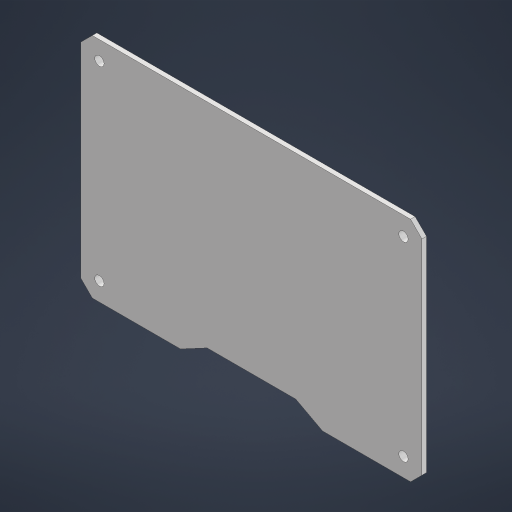
# Autodesk Inventor part: Top
Saved by Autodesk Inventor 2024.2 (Build 282272000, 272)
## iProperties
Created: 2024-06-04
Part Number: Top
Material: Generic
Document SubType Name: Modeling
Designer: simon
Density: 1 g/cm^3
Appearance: Default
Author: simon
Autodesk Inventor part; units mm, degrees
ref_plane "YZ Plane" through (0, 0, 0) normal (1, 0, 0) x (0, 1, 0)
ref_plane "XZ Plane" through (0, 0, 0) normal (0, 1, 0) x (-1, 0, 0)
ref_plane "XY Plane" through (0, 0, 0) normal (0, 0, 1) x (1, 0, 0)
sketch "Sketch1" plane through (0, 0, 0) normal (0, 0, 1) x (1, 0, 0)
  line L0 (0, 0) -> (120, 0)
  line L1 (120, 0) -> (120, 80)
  line L2 (120, 80) -> (0, 80)
  line L3 (0, 80) -> (0, 0)
  line L4 (114.4, 1.6) -> (85, 1.6) projected
  line L5 (75.6, 6.6) -> (85, 1.6) projected
  line L6 (44.4, 6.6) -> (75.6, 6.6) projected
  line L7 (35, 1.6) -> (44.4, 6.6) projected
  line L8 (35, 1.6) -> (5.6, 1.6) projected
  line L9 (1.6, 5.6) -> (5.6, 1.6) projected
  line L10 (1.6, 5.6) -> (1.6, 74.4) projected
  line L11 (5.6, 78.4) -> (1.6, 74.4) projected
  line L12 (5.6, 78.4) -> (114.4, 78.4) projected
  line L13 (118.4, 74.4) -> (114.4, 78.4) projected
  line L14 (118.4, 74.4) -> (118.4, 5.6) projected
  line L15 (114.4, 1.6) -> (118.4, 5.6) projected
  line L16 (116, 80) -> (120, 76) projected
  line L17 (116, 80) -> (4, 80) projected
  line L18 (0, 76) -> (4, 80) projected
  line L19 (0, 76) -> (0, 4) projected
  line L20 (4, 0) -> (0, 4) projected
  line L21 (4, 0) -> (35, 0) projected
  line L22 (44.4, 5) -> (35, 0) projected
  line L23 (44.4, 5) -> (75.6, 5) projected
  line L24 (75.6, 5) -> (85, 0) projected
  line L25 (85, 0) -> (116, 0) projected
  line L26 (120, 4) -> (116, 0) projected
  line L27 (120, 4) -> (120, 76) projected
  circle A0 centre (6.5, 73.5) radius 2 projected
  circle A1 centre (6.5, 6.5) radius 2 projected
  circle A2 centre (113.5, 6.5) radius 2 projected
  circle A3 centre (113.5, 73.5) radius 2 projected
  circle A4 centre (6.5, 73.5) radius 1.65
  circle A5 centre (113.5, 73.5) radius 1.65
  circle A6 centre (113.5, 6.5) radius 1.65
  circle A7 centre (6.5, 6.5) radius 1.65
  line L28 (0, 4) -> (4, 0)
  line L29 (0, 76) -> (4, 80)
  line L30 (116, 80) -> (120, 76)
  line L31 (116, 0) -> (120, 4)
  line L32 (35, 0) -> (44.4, 5)
  line L33 (44.4, 5) -> (75.6, 5)
  line L34 (75.6, 5) -> (85, 0)
  dimension "d0" = 120
  dimension "d1" = 80
  dimension "d4" = 3.3
  dimension "d5" = 3.3
  dimension "d6" = 3.3
  dimension "d7" = 3.3
  constraints: 22 end point, 7 equal length, 4 centre point, 4 coincident, 2 perpendicular, 1 horizontal, 1 point on line
  measures "d0" distance of L2.end L1.end
  measures "d1" distance of L1.end L0.end
  measures "d4" diameter of A4
  measures "d5" diameter of A5
  measures "d6" diameter of A6
  measures "d7" diameter of A7
extrude "Extrusion1" add sketch "Sketch1" along normal blind 1.6 contours L20 L3 L18 L2 L16 L1 L26 L0 L24 L23 L22 | L4 L5 L6 L7 L8 L9 L10 L11 L12 L13 L14 L15 | A0 | A1 | A2 | A3
sketch "Sketch2" plane through (0, 0, 1.6) normal (0, 0, 1) x (1, 0, 0)
  line L0 (5.6, 78.4) -> (114.4, 78.4) projected
  line L1 (5.6, 78.4) -> (1.6, 74.4) projected
  line L2 (1.6, 5.6) -> (1.6, 74.4) projected
  circle A0 centre (6.5, 73.5) radius 2 projected
  circle A1 centre (6.5, 6.5) radius 2 projected
  line L3 (1.6, 5.6) -> (5.6, 1.6) projected
  line L4 (16.9137, 1.6) -> (1.6, 16.9137) projected
  line L5 (35, 1.6) -> (5.6, 1.6) projected
  line L6 (35, 1.6) -> (44.4, 6.6) projected
  line L7 (44.4, 6.6) -> (75.6, 6.6) projected
  line L8 (75.6, 6.6) -> (85, 1.6) projected
  line L9 (114.4, 1.6) -> (85, 1.6) projected
  line L10 (114.4, 1.6) -> (118.4, 5.6) projected
  line L11 (118.4, 74.4) -> (118.4, 5.6) projected
  line L12 (118.4, 16.9137) -> (103.0863, 1.6) projected
  circle A2 centre (113.5, 6.5) radius 2 projected
  line L13 (103.0863, 78.4) -> (118.4, 63.0863) projected
  circle A3 centre (113.5, 73.5) radius 2 projected
  line L14 (114.4, 78.4) -> (118.4, 74.4) projected
  line L15 (1.6, 63.0863) -> (16.9137, 78.4) projected
  circle A4 centre (6.5, 73.5) radius 2 projected
  line L16 (118.2, 5.6828) -> (114.3172, 1.8)
  line L17 (114.3172, 1.8) -> (85.0499, 1.8)
  line L18 (85.0499, 1.8) -> (75.6499, 6.8)
  line L19 (75.6499, 6.8) -> (44.3501, 6.8)
  line L20 (44.3501, 6.8) -> (34.9501, 1.8)
  line L21 (34.9501, 1.8) -> (5.6828, 1.8)
  line L22 (5.6828, 1.8) -> (1.8, 5.6828)
  line L23 (1.8, 5.6828) -> (1.8, 74.3172)
  line L24 (1.8, 74.3172) -> (5.6828, 78.2)
  line L25 (5.6828, 78.2) -> (114.3172, 78.2)
  line L26 (114.3172, 78.2) -> (118.2, 74.3172)
  line L27 (118.2, 74.3172) -> (118.2, 5.6828)
  line L28 (75.6, 5) -> (85, 0) projected
  line L29 (118.2, 16.7137) -> (103.2863, 1.8)
  line L30 (16.7137, 1.8) -> (1.8, 16.7137)
  line L31 (1.8, 63.2863) -> (16.7137, 78.2)
  line L32 (103.2863, 78.2) -> (118.2, 63.2863)
  circle A5 centre (113.5, 6.5) radius 1.65
  circle A6 centre (113.5, 73.5) radius 1.65
  circle A7 centre (6.5, 73.5) radius 1.65
  circle A8 centre (6.5, 6.5) radius 1.65
  line L33 (104.0863, 2.6) -> (85.2494, 2.6)
  line L34 (85.2494, 2.6) -> (75.8494, 7.6)
  line L35 (75.8494, 7.6) -> (44.1506, 7.6)
  line L36 (44.1506, 7.6) -> (34.7506, 2.6)
  line L37 (34.7506, 2.6) -> (15.9137, 2.6)
  line L38 (2.6, 15.9137) -> (2.6, 64.0863)
  line L39 (15.9137, 77.4) -> (104.0863, 77.4)
  line L40 (117.4, 64.0863) -> (117.4, 15.9137)
  point P0 (0, 0)
  dimension "d9" = 0.2
  dimension "d10" = 0.2
  dimension "d11" = 0.2
  dimension "d12" = 0.2
  dimension "d13" = 0.2
  dimension "d14" = 0.2
  dimension "d15" = 0.2
  dimension "d16" = 0.2
  dimension "d17" = 0.2
  dimension "d18" = 0.2
  dimension "d19" = 0.2
  dimension "d21" = 0.2
  dimension "d22" = 3.3
  dimension "d23" = 3.3
  dimension "d24" = 3.3
  dimension "d25" = 3.3
  dimension "d26" = 0.8
  dimension "d27" = 0.8
  dimension "d28" = 0.8
  dimension "d29" = 0.8
  dimension "d30" = 0.8
  dimension "d31" = 0.8
  dimension "d32" = 0.8
  dimension "d33" = 0.8
  constraints: 48 end point, 24 point on line, 20 parallel, 4 centre point, 4 coincident, 2 horizontal, 2 perpendicular, 1 collinear
  measures "d9" distance between parallel lines of L9 L17
  measures "d10" distance between parallel lines of L10 L16
  measures "d11" distance between parallel lines of L11 L27
  measures "d12" distance between parallel lines of L14 L26
  measures "d13" distance between parallel lines of L0 L25
  measures "d14" distance between parallel lines of L1 L24
  measures "d15" distance between parallel lines of L2 L23
  measures "d16" distance between parallel lines of L3 L22
  measures "d17" distance between parallel lines of L5 L21
  measures "d18" distance between parallel lines of L6 L20
  measures "d19" distance between parallel lines of L7 L19
  measures "d21" distance between parallel lines of L8 L18
  measures "d22" diameter of A5
  measures "d23" diameter of A6
  measures "d24" diameter of A7
  measures "d25" diameter of A8
  measures "d26" distance between parallel lines of L17 L33
  measures "d27" distance between parallel lines of L18 L34
  measures "d28" distance between parallel lines of L19 L35
  measures "d29" distance between parallel lines of L20 L36
  measures "d30" distance between parallel lines of L21 L37
  measures "d31" distance between parallel lines of L38 L23
  measures "d32" distance between parallel lines of L39 L25
  measures "d33" distance between parallel lines of L40 L27
extrude "Extrusion2" add sketch "Sketch2" against normal blind 3.2 contours L25 L13 L39 L15 | L15 L23 L24 L25 | L25 L26 L27 L13 | L15 L38 L4 L23 | L4 L21 L22 L23 | L13 L27 L12 L40 | L12 L27 L16 L17 | L37 L36 L35 L34 L33 L12 L17 L18 L19 L20 L21 L4 | A0 | A1 | A2 | A3
body "Solid1"
